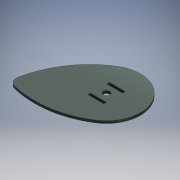
# Autodesk Inventor part: leva00
Saved by Autodesk Inventor 2016 (Build 200138000, 138)
## iProperties
Created: 2016-09-20
Part Number: leva00
Material: Madera (abedul)
Document SubType Name: Modeling
Designer: i95sa
Density: 0.55 g/cm^3
Appearance: Gris plomo - Pulido
Author: i95sa
Autodesk Inventor part; units mm, degrees
ref_plane "YZ Plane" through (0, 0, 0) normal (1, 0, 0) x (0, 1, 0)
ref_plane "XZ Plane" through (0, 0, 0) normal (0, 1, 0) x (-1, 0, 0)
ref_plane "XY Plane" through (0, 0, 0) normal (0, 0, 1) x (1, 0, 0)
sketch "Boceto1" plane through (0, 0, 0) normal (0, 0, 1) x (1, 0, 0)
  arc A0 (44.5087, 28.2461) -> (-44.5087, -28.2461) centre (0, 0) ccw
  arc A1 (-68.4955, -43.4685) -> (-89.038, -56.5052) centre (-78.7667, -49.9869) ccw
  line L0 (-92.0117, -58.3924) -> (-98.5301, -48.1212)
  line L1 (-27.7169, 44.8402) -> (-38.5808, 61.959)
  line L2 (-38.5808, 61.959) -> (-98.5301, -48.1212)
  line L3 (-98.5301, -48.1212) -> (-75.2574, -5.3874)
  arc A2 (-27.7169, 44.8402) -> (-75.2574, -5.3874) centre (43.2095, -69.9041) ccw
  arc A3 (-75.2574, -5.3874) -> (-90.682, -47.5346) centre (58.5185, -78.2413) ccw
  line L4 (3.4237, 2.1728) -> (44.5087, 28.2461)
  line L5 (-3.4237, -2.1728) -> (-92.0117, -58.3924)
  arc A4 (-44.5087, -28.2461) -> (44.5087, 28.2461) centre (0, 0) ccw
  arc A5 (-89.038, -56.5052) -> (-68.4955, -43.4685) centre (-78.7667, -49.9869) ccw
  line L6 (-92.0117, -58.3924) -> (-85.4934, -68.6637)
  line L7 (28.7714, -44.171) -> (39.6353, -61.2898)
  line L8 (39.6353, -61.2898) -> (-85.4934, -68.6637)
  line L9 (-85.4934, -68.6637) -> (-36.9177, -65.8011)
  arc A6 (-36.9177, -65.8011) -> (28.7714, -44.171) centre (-44.8534, 68.8608) ccw
  arc A7 (-81.6211, -61.8123) -> (-36.9177, -65.8011) centre (-45.8789, 86.2627) ccw
  dimension "d0" = 105.43
  dimension "d6" = 24.33
  dimension "d7" = 12.165
  dimension "d8" = 20.275
  dimension "d9" = 48.66
  constraints: 20 end point, 20 point on circle, 8 centre point, 6 symmetric about line, 5 point on line, 4 tangent, 1 collinear, 4 other
  measures "d0" diameter of A0
  measures "d6" diameter of A1
  measures "d7" distance of L0.start L0.end
  measures "d8" distance of L1.start L1.end
  measures "d9" distance of L0.end L3.end
extrude "Extrusión2" add sketch "Boceto1" along normal blind 4 contours A4 A0 | A0 L5 A1 A3 A2 | A6 A7 A5 L5 A4 | L5 A1 | A5 L5
sketch "Boceto2" plane through (0, 0, 4) normal (0, 0, 1) x (1, 0, 0)
  line L0 (0, 0) -> (0, 12.5)
  line L1 (0, 12.5) -> (-12.5, 12.5)
  line L2 (-12.5, 12.5) -> (-12.5, 16.7)
  line L3 (-12.5, 16.7) -> (12.5, 16.7)
  line L4 (12.5, 16.7) -> (12.5, 12.5)
  line L5 (12.5, 12.5) -> (0, 12.5)
  line L6 (0, 0) -> (12.5, 0)
  line L7 (0, 0) -> (0, -12.5)
  line L8 (0, -12.5) -> (-12.5, -12.5)
  line L9 (-12.5, -12.5) -> (-12.5, -16.7)
  line L10 (-12.5, -16.7) -> (12.5, -16.7)
  line L11 (12.5, -16.7) -> (12.5, -12.5)
  line L12 (12.5, -12.5) -> (0, -12.5)
  circle A0 centre (0, 0) radius 5
  dimension "d24" = 12.5
  dimension "d25" = 12.5
  dimension "d26" = 4.2
  dimension "d27" = 25
  dimension "d28" = 10
  constraints: 26 end point, 5 perpendicular, 5 symmetric about line, 3 point on line, 1 centre point, 1 coincident, 1 parallel, 1 vertical
  measures "d24" distance of L0.start L0.end
  measures "d25" distance of L0.end L1.end
  measures "d26" distance of L1.end L2.end
  measures "d27" distance of L2.end L3.end
  measures "d28" diameter of A0
extrude "Extrusión3" cut sketch "Boceto2" against normal blind 4
